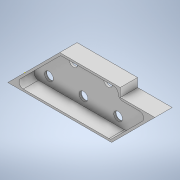
# Autodesk Inventor part: Ch4 Part 1
Saved by Autodesk Inventor 2020 (Build 240168000, 168)
## iProperties
Created: 2021-02-05
Part Number: Ch4 Part 1
Material: Generic
Document SubType Name: Modeling
Designer: austi
Density: 1 g/cm^3
Appearance: Default
Author: austi
Autodesk Inventor part; units mm, degrees
ref_plane "YZ Plane" through (0, 0, 0) normal (1, 0, 0) x (0, 1, 0)
ref_plane "XZ Plane" through (0, 0, 0) normal (0, 1, 0) x (-1, 0, 0)
ref_plane "XY Plane" through (0, 0, 0) normal (0, 0, 1) x (1, 0, 0)
sketch "Sketch1" plane through (0, 0, 0) normal (0, 0, 1) x (1, 0, 0)
  line L0 (-21.59, 0) -> (129.54, 0) projected
  line L1 (0, -7.62) -> (0, 45.72) projected
  line L2 (0, 0) -> (38.1, 38.1)
  line L3 (38.1, 38.1) -> (82.55, 38.1)
  line L4 (82.55, 38.1) -> (82.55, 31.75)
  line L5 (82.55, 31.75) -> (107.95, 31.75)
  line L6 (107.95, 31.75) -> (76.2, 0)
  line L7 (0, 0) -> (76.2, 0)
  dimension "d0" = 38.1
  dimension "d1" = 45
  dimension "d2" = 76.2
  dimension "d3" = 25.4
  dimension "d27" = 6.35
  constraints: 12 end point, 2 perpendicular, 2 point on line, 1 coincident, 1 collinear, 1 horizontal, 1 horizontal alignment, 1 parallel
  measures "d0" horizontal distance of L2.end point (0, 0)
  measures "d1" angle of L0 L6
  measures "d2" distance of L2.start L6.end
  measures "d3" distance of L4.end L5.end
  measures "d27" distance of L3.end L4.end
sketch "Sketch2" plane through (0, 0, 0) normal (0, 0, 1) x (1, 0, 0)
  point P0 (0, 0)
extrude "Extrusion1" add sketch "Sketch1" along normal blind 12.7
shell "Shell1" thickness 1.524 removed faces 1 at (38.1, 12.7, 12.7)
fillet "Fillet1" radius 3.175 6 edges at (38.7313, 36.576, 7.112) (81.026, 36.576, 7.112) (81.026, 30.226, 7.112) (104.2707, 30.226, 7.112) (75.5687, 1.524, 7.112) (3.6793, 1.524, 7.112)
sketch "Sketch3" plane through (11.3444, 1.524, 1.524) normal (0, 0, 1) x (1, 0, 0)
  line L0 (-11.3444, -1.524) -> (64.8556, -1.524) projected
  line L1 (-11.3444, -1.524) -> (7.7056, -1.524)
  line L2 (7.7056, -1.524) -> (7.7056, 6.35)
  circle A0 centre (7.7056, 6.35) radius 3.175
  line L3 (7.7056, 6.35) -> (25.6661, 24.3105) construction
  line L4 (-2.2451, 5.4201) -> (26.4569, 34.1221) projected
  circle A1 centre (25.6661, 24.3105) radius 3.175
  circle A2 centre (33.1056, 6.35) radius 3.175
  circle A3 centre (58.5056, 6.35) radius 3.175
  circle A4 centre (51.0661, 24.3105) radius 3.175
  circle A5 centre (76.4661, 24.3105) radius 3.175
  dimension "d32" = 19.05
  dimension "d33" = 7.874
  dimension "d35" = 25.4
  dimension "d41" = 25.4
  dimension "d42" = 25.4
  dimension "d46" = 6.35
  dimension "d47" = 25.4
  dimension "d48" = 25.4
  constraints: 6 centre point, 6 end point, 5 equal radius, 5 horizontal alignment, 2 coincident, 1 parallel, 1 perpendicular, 1 point on line
  measures "d32" distance of L0.start L1.end
  measures "d33" distance of L1.end L2.end
  measures "d35" distance of L3.start L3.end
  measures "d41" distance of A2.centre L2.end
  measures "d42" distance of A3.centre A2.centre
  measures "d46" diameter of A4
  measures "d47" distance of A4.centre L3.end
  measures "d48" distance of A5.centre A4.centre
extrude "Extrusion2" cut sketch "Sketch3" against normal through all
body "Solid1"
